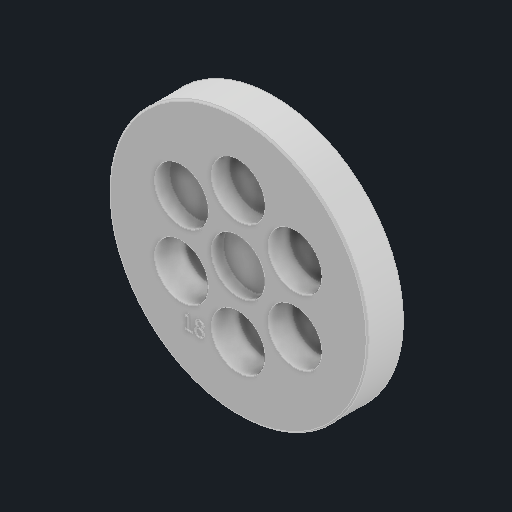
# Autodesk Inventor part: Diameter_18mm
Saved by Autodesk Inventor 2026 (Build 300175050, 175E)
## iProperties
Created: 2023-09-28
Part Number: Diameter_18mm
Material: Generic
Document SubType Name: Modeling
Designer: Konstantin
Density: 1 g/cm^3
Appearance: Default
Author: Konstantin
Autodesk Inventor part; units mm, degrees
ref_plane "YZ Plane" through (0, 0, 0) normal (1, 0, 0) x (0, 1, 0)
ref_plane "XZ Plane" through (0, 0, 0) normal (0, 1, 0) x (-1, 0, 0)
ref_plane "XY Plane" through (0, 0, 0) normal (0, 0, 1) x (1, 0, 0)
sketch "Sketch1" plane through (0, 0, 0) normal (0, 0, 1) x (1, 0, 0)
  circle A0 centre (0, 0) radius 43.5
  circle A1 centre (0, 0) radius 9
  circle A2 centre (0, 22) radius 9
  circle A3 centre (-19.0526, 11) radius 9
  circle A4 centre (-19.0526, -11) radius 9
  circle A5 centre (0, -22) radius 9
  circle A6 centre (19.0526, -11) radius 9
  circle A7 centre (19.0526, 11) radius 9
  dimension "diameter" = 18
  dimension "d2" = 18
  dimension "d5" = 360
  dimension "d7" = 22
  dimension "d28" = 87
  constraints: 8 centre point, 2 coincident, 13 other
  measures "diameter" diameter of A1
  measures "d2" diameter of A2
  measures "d7" distance of point (0, 0) A2.centre
  measures "d28" diameter of A0
extrude "Extrusion1" add sketch "Sketch1" along normal blind 12
sketch "Sketch2" plane through (0, 0, 12) normal (0, 0, 1) x (1, 0, 0)
  line L0 (-5.8774, 39.105) -> (5.7366, 39.105) construction
  line L1 (5.7366, 39.105) -> (5.7366, 35.936) construction
  line L2 (5.7366, 35.936) -> (-5.8774, 35.936) construction
  line L3 (-5.8774, 35.936) -> (-5.8774, 39.105) construction
  point P0 (0, 0)
  constraints: 2 other
emboss "Emboss1" [suppressed]
chamfer "Chamfer1" distance 0.5 angle 45 1 edges at (-43.5, 0, 12)
extrude "Extrusion11" add sketch "Sketch1" along normal blind 2 contours A4
extrude "Extrusion12" add sketch "Sketch1" along normal blind 3 contours A5
extrude "Extrusion13" add sketch "Sketch1" along normal blind 4 contours A6
extrude "Extrusion14" add sketch "Sketch1" along normal blind 5 contours A7
extrude "Extrusion15" add sketch "Sketch1" along normal blind 6 contours A2
extrude "Extrusion16" add sketch "Sketch1" along normal blind 7 contours A3
extrude "Extrusion17" add sketch "Sketch1" along normal blind 8 contours A1
sketch "Skizze3" plane through (0, 0, 12) normal (0, 0, 1) x (1, 0, 0)
  line L0 (-4.3129, -31.1582) -> (0.2616, -31.1582) construction
  line L1 (0.2616, -31.1582) -> (0.2616, -34.3322) construction
  line L2 (0.2616, -34.3322) -> (-4.3129, -34.3322) construction
  line L3 (-4.3129, -34.3322) -> (-4.3129, -31.1582) construction
  line L4 (28.3417, 16.1952) -> (30.6289, 16.1952) construction
  line L5 (30.6289, 16.1952) -> (30.6289, 13.0262) construction
  line L6 (30.6289, 13.0262) -> (28.3417, 13.0262) construction
  line L7 (28.3417, 13.0262) -> (28.3417, 16.1952) construction
  line L8 (-27.2854, 19.1878) -> (-24.9982, 19.1878) construction
  line L9 (-24.9982, 19.1878) -> (-24.9982, 16.0015) construction
  line L10 (-24.9982, 16.0015) -> (-27.2854, 16.0015) construction
  line L11 (-27.2854, 16.0015) -> (-27.2854, 19.1878) construction
  line L12 (-18.5838, -22.0358) -> (-14.0094, -22.0358) construction
  line L13 (-14.0094, -22.0358) -> (-14.0094, -25.2048) construction
  line L14 (-14.0094, -25.2048) -> (-18.5838, -25.2048) construction
  line L15 (-18.5838, -25.2048) -> (-18.5838, -22.0358) construction
  line L16 (-11.1833, -16.7575) -> (-8.896, -16.7575) construction
  line L17 (-8.896, -16.7575) -> (-8.896, -19.8055) construction
  line L18 (-8.896, -19.8055) -> (-11.1833, -19.8055) construction
  line L19 (-11.1833, -19.8055) -> (-11.1833, -16.7575) construction
  line L20 (20.4292, 1.4865) -> (22.7164, 1.4865) construction
  line L21 (22.7164, 1.4865) -> (22.7164, -1.6825) construction
  line L22 (22.7164, -1.6825) -> (20.4292, -1.6825) construction
  line L23 (20.4292, -1.6825) -> (20.4292, 1.4865) construction
  line L24 (-11.5764, 19.8878) -> (-9.2892, 19.8878) construction
  line L25 (-9.2892, 19.8878) -> (-9.2892, 16.7756) construction
  line L26 (-9.2892, 16.7756) -> (-11.5764, 16.7756) construction
  line L27 (-11.5764, 16.7756) -> (-11.5764, 19.8878) construction
  line L28 (3.9152, 10.1367) -> (6.2025, 10.1367) construction
  line L29 (6.2025, 10.1367) -> (6.2025, 7.0887) construction
  line L30 (6.2025, 7.0887) -> (3.9152, 7.0887) construction
  line L31 (3.9152, 7.0887) -> (3.9152, 10.1367) construction
  line L32 (-15.3869, -27.1492) -> (-17.8261, -27.1492)
  line L33 (-17.8261, -27.1492) -> (-17.8261, -26.6387)
  line L34 (-17.8261, -26.6387) -> (-16.9185, -26.6387)
  line L35 (-16.9185, -26.6387) -> (-16.9185, -23.2878)
  line L36 (-16.9185, -23.2878) -> (-17.8261, -23.2878)
  line L37 (-17.8261, -23.2878) -> (-17.8261, -22.8299)
  spline S0 degree 2 poles (-17.8261, -22.8299) (-17.3115, -22.8299) (-16.8253, -22.5382) (-16.7929, -22.133) knots 0 0 0 1 2 2 2
  line L38 (-16.7929, -22.133) -> (-16.2743, -22.133)
  line L39 (-16.2743, -22.133) -> (-16.2743, -26.6387)
  line L40 (-16.2743, -26.6387) -> (-15.3869, -26.6387)
  line L41 (-15.3869, -26.6387) -> (-15.3869, -27.1492)
  spline S1 degree 2 poles (-12.9558, -27.2627) (-13.3286, -27.2627) (-13.9404, -27.0398) (-14.1551, -26.8332) knots 0 0 0 1 2 2 2
  spline S2 degree 2 poles (-14.1551, -26.8332) (-14.3658, -26.6306) (-14.5846, -26.0795) (-14.5846, -25.7675) knots 0 0 0 1 2 2 2
  spline S3 degree 2 poles (-14.5846, -25.7675) (-14.5846, -25.3623) (-14.1511, -24.6816) (-13.7378, -24.479) knots 0 0 0 1 2 2 2
  line L42 (-13.7378, -24.479) -> (-13.7378, -24.4588)
  spline S4 degree 2 poles (-13.7378, -24.4588) (-14.1065, -24.244) (-14.4631, -23.7335) (-14.4631, -23.3526) knots 0 0 0 1 2 2 2
  spline S5 degree 2 poles (-14.4631, -23.3526) (-14.4631, -22.7894) (-13.6122, -22.0358) (-12.9558, -22.0358) knots 0 0 0 1 2 2 2
  spline S6 degree 2 poles (-12.9558, -22.0358) (-12.2751, -22.0358) (-11.4525, -22.7489) (-11.4525, -23.308) knots 0 0 0 1 2 2 2
  spline S7 degree 2 poles (-11.4525, -23.308) (-11.4525, -23.6444) (-11.8456, -24.3008) (-12.2143, -24.4871) knots 0 0 0 1 2 2 2
  line L43 (-12.2143, -24.4871) -> (-12.2143, -24.5074)
  spline S8 degree 2 poles (-12.2143, -24.5074) (-11.7767, -24.71) (-11.3269, -25.2935) (-11.3269, -25.7554) knots 0 0 0 1 2 2 2
  spline S9 degree 2 poles (-11.3269, -25.7554) (-11.3269, -26.3956) (-12.2589, -27.2627) (-12.9558, -27.2627) knots 0 0 0 1 2 2 2
  spline S10 degree 2 poles (-12.0158, -25.8202) (-12.0158, -25.5123) (-12.2589, -25.1476) (-12.6033, -24.9612) knots 0 0 0 1 2 2 2
  spline S11 degree 2 poles (-12.6033, -24.9612) (-12.7167, -24.8964) (-13.0976, -24.7465) (-13.3367, -24.6492) knots 0 0 0 1 2 2 2
  spline S12 degree 2 poles (-13.3367, -24.6492) (-13.6122, -24.8315) (-13.908, -25.3745) (-13.908, -25.7189) knots 0 0 0 1 2 2 2
  spline S13 degree 2 poles (-13.908, -25.7189) (-13.908, -26.1727) (-13.361, -26.7643) (-12.9477, -26.7643) knots 0 0 0 1 2 2 2
  spline S14 degree 2 poles (-12.9477, -26.7643) (-12.5263, -26.7643) (-12.0158, -26.2578) (-12.0158, -25.8202) knots 0 0 0 1 2 2 2
  spline S15 degree 2 poles (-12.1089, -23.3162) (-12.1089, -22.9798) (-12.5587, -22.5301) (-12.9598, -22.5301) knots 0 0 0 1 2 2 2
  spline S16 degree 2 poles (-12.9598, -22.5301) (-13.3245, -22.5301) (-13.7905, -22.9312) (-13.7905, -23.2756) knots 0 0 0 1 2 2 2
  spline S17 degree 2 poles (-13.7905, -23.2756) (-13.7905, -23.5228) (-13.5514, -23.8672) (-13.3123, -24.005) knots 0 0 0 1 2 2 2
  spline S18 degree 2 poles (-13.3123, -24.005) (-13.2111, -24.0617) (-12.7816, -24.2602) (-12.6073, -24.317) knots 0 0 0 1 2 2 2
  spline S19 degree 2 poles (-12.6073, -24.317) (-12.3156, -24.0941) (-12.1089, -23.62) (-12.1089, -23.3162) knots 0 0 0 1 2 2 2
  point P0 (0, 0)
  constraints: 16 other
emboss "Prägen2" sketch "Skizze3" operation cut depth 0.6 direction (0, 0, -1)
sketch "Skizze4" plane through (0, 0, 12) normal (0, 0, 1) x (1, 0, 0)
  circle A0 centre (0, 0) radius 40.5
  circle A1 centre (0, 0) radius 35
  dimension "d58" = 81
  dimension "d59" = 70
  constraints: 2 centre point, 2 coincident
  measures "d58" diameter of A0
  measures "d59" diameter of A1
extrude "Extrusion18" [suppressed]
equation "\"d2\" = diameter"
body "Solid1"
